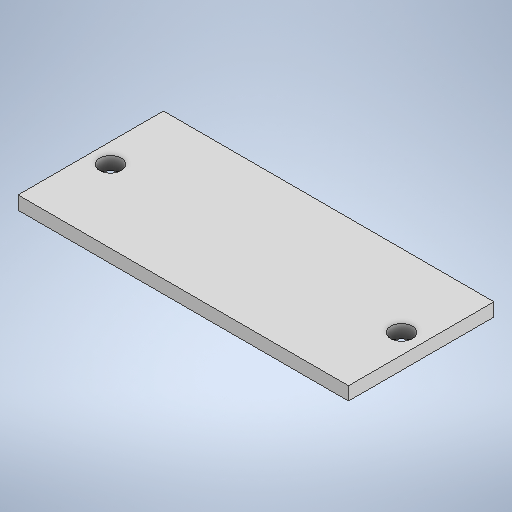
# Autodesk Inventor part: IMU_shin_mount_clamp
Saved by Autodesk Inventor 2025.2 (Build 292293000, 293)
## iProperties
Created: 2025-01-16
Part Number: IMU_shin_mount_clamp
Material: Generic
Document SubType Name: Modeling
Designer: email
Density: 1 g/cm^3
Appearance: Default
Author: email
Autodesk Inventor part; units mm, degrees
ref_plane "YZ Plane" through (0, 0, 0) normal (1, 0, 0) x (0, 1, 0)
ref_plane "XZ Plane" through (0, 0, 0) normal (0, 1, 0) x (-1, 0, 0)
ref_plane "XY Plane" through (0, 0, 0) normal (0, 0, 1) x (1, 0, 0)
sketch "Sketch1" plane through (0, 0, 0) normal (0, 1, 0) x (-1, 0, 0)
  line L0 (25, -22) -> (25, 0)
  line L1 (-25, 0) -> (25, 0)
  line L2 (25, -22) -> (19.05, -22)
  line L3 (19.05, 0) -> (25, 0)
  line L4 (25, 0) -> (25, -22)
  line L5 (-25, -22) -> (-19.05, -22)
  line L6 (-19.05, 0) -> (-25, 0)
  line L7 (-25, 0) -> (-25, -22)
  circle A0 centre (22.025, -11) radius 1.65
  circle A1 centre (-22.025, -11) radius 1.65
  line L8 (25, 0) -> (-25, 0)
  line L9 (-25, 0) -> (-25, -22)
  line L10 (-25, -22) -> (25, -22)
  line L11 (25, -22) -> (25, 0)
  point P0 (0, 0)
  point P1 (22.025, 0)
  point P2 (-25, -11)
  point P3 (0, 0)
  dimension "d2" = 3.3
  dimension "d3" = 3.3
  dimension "d4" = 2.975
  dimension "d5" = 11
  dimension "d6" = 2.975
  dimension "d7" = 11
  constraints: 24 end point, 4 parallel, 3 horizontal, 3 midpoint, 2 centre point, 2 point on line, 1 coincident, 1 perpendicular
  measures "d2" diameter of A0
  measures "d3" diameter of A1
  measures "d4" distance from line of L0 A0.centre
  measures "d5" distance of point (22.025, 0) A0.centre
  measures "d6" distance of point (-25, -11) A1.centre
  measures "d7" distance from line of L1 A1.centre
extrude "Extrusion1" add sketch "Sketch1" along normal blind 2
body "Solid1"
